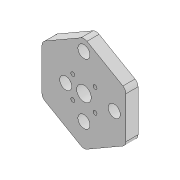
# Autodesk Inventor part: Flange
Saved by Autodesk Inventor 2020 (Build 240168000, 168)
## iProperties
Created: 2021-08-17
Part Number: Flange
Material: 一般
Document SubType Name: Modeling
Designer: ken113
Density: 1 g/cm^3
Appearance: 既定
Author: ken113
Autodesk Inventor part; units mm, degrees
ref_plane "YZ Plane" through (0, 0, 0) normal (1, 0, 0) x (0, 1, 0)
ref_plane "XZ Plane" through (0, 0, 0) normal (0, 1, 0) x (-1, 0, 0)
ref_plane "XY Plane" through (0, 0, 0) normal (0, 0, 1) x (1, 0, 0)
sketch "スケッチ1" plane through (0, 0, 0) normal (0, 0, 1) x (1, 0, 0)
  line L0 (0, 40) -> (34.641, 20)
  line L1 (34.641, 20) -> (34.641, -20)
  line L2 (34.641, -20) -> (0, -40)
  line L3 (0, -40) -> (-34.641, -20)
  line L4 (-34.641, -20) -> (-34.641, 20)
  line L5 (-34.641, 20) -> (0, 40)
  point P0 (0, 0)
  point P1 (0, 0)
  dimension "d0" = 40
  constraints: 12 end point, 1 coincident, 1 vertical alignment, 13 other
  measures "d0" distance of point (0, 0) L0.start
extrude "押し出し1" add sketch "スケッチ1" along normal blind 10
sketch "スケッチ2" plane through (0, 0, 10) normal (0, 0, 1) x (1, 0, 0)
  line L0 (0, -40) -> (34.641, -20) projected
  line L1 (34.641, -20) -> (34.641, 20) projected
  line L2 (34.641, 20) -> (0, 40) projected
  line L3 (0, 40) -> (-34.641, 20) projected
  line L4 (-34.641, 20) -> (-34.641, -20) projected
  line L5 (-34.641, -20) -> (0, -40) projected
  point P0 (0, 0)
  point P1 (0, 30)
  point P2 (25, 0)
  point P3 (0, -20)
  point P4 (-15, 0)
  dimension "d3" = 30
  dimension "d4" = 25
  dimension "d5" = 20
  dimension "d6" = 15
  measures "d3" distance of point (0, 30) point (0, 0)
  measures "d4" distance of point (25, 0) point (0, 0)
  measures "d5" distance of point (0, -20) point (0, 0)
  measures "d6" distance of point (0, 0) point (-15, 0)
hole "穴1" at (0, 30, 10) at (25, 0, 10) at (0, -20, 10) at (-15, 0, 10) direction (0, 0, -1) diameter 4.2 depth 10 counterbore diameter 10 counterbore depth 7
sketch "スケッチ3" plane through (0, 0, 0) normal (0, 0, -1) x (-1, 0, 0)
  circle A0 centre (0, -20) radius 2.1 projected
  circle A1 centre (0, 30) radius 2.1 projected
  circle A2 centre (-25, 0) radius 2.1 projected
  circle A3 centre (15, 0) radius 2.1 projected
  line L0 (0, -40) -> (-34.641, -20) projected
  line L1 (34.641, -20) -> (0, -40) projected
  line L2 (34.641, 20) -> (34.641, -20) projected
  line L3 (0, 40) -> (34.641, 20) projected
  line L4 (-34.641, 20) -> (0, 40) projected
  line L5 (-34.641, -20) -> (-34.641, 20) projected
  circle A4 centre (0, 0) radius 13
  point P0 (9.1924, -9.1924)
  point P1 (9.1924, 9.1924)
  point P2 (-9.1924, 9.1924)
  point P3 (-9.1924, -9.1924)
  dimension "d14" = 26
  dimension "d17" = 360
  constraints: 1 coincident, 1 horizontal alignment, 8 other
hole "穴2" at (-9.1924, -9.1924, 0) at (-9.1924, 9.1924, 0) at (9.1924, 9.1924, 0) at (9.1924, -9.1924, 0) direction (0, 0, 1) diameter 3.242 depth 12 thread size "M4x0.7" class "6H" standard "ISO Metric profile"
sketch "スケッチ4" plane through (0, 0, 0) normal (0, 0, -1) x (-1, 0, 0)
  circle A0 centre (-9.1924, 9.1924) radius 1.621 projected
  circle A1 centre (9.1924, -9.1924) radius 1.621 projected
  circle A2 centre (9.1924, 9.1924) radius 1.621 projected
  circle A3 centre (-9.1924, -9.1924) radius 1.621 projected
  circle A4 centre (0, -20) radius 2.1 projected
  circle A5 centre (0, 30) radius 2.1 projected
  circle A6 centre (-25, 0) radius 2.1 projected
  circle A7 centre (15, 0) radius 2.1 projected
  line L0 (0, -40) -> (-34.641, -20) projected
  line L1 (34.641, -20) -> (0, -40) projected
  line L2 (34.641, 20) -> (34.641, -20) projected
  line L3 (0, 40) -> (34.641, 20) projected
  line L4 (-34.641, 20) -> (0, 40) projected
  line L5 (-34.641, -20) -> (-34.641, 20) projected
  point P0 (0, 0)
hole "穴3" at (0, 30, 0) at (-15, 0, 0) at (0, -20, 0) at (25, 0, 0) direction (0, 0, 1) diameter 5.5 depth 12 countersink diameter 10.6 countersink angle 90
sketch "スケッチ5" plane through (0, 0, 0) normal (0, 0, -1) x (-1, 0, 0)
  circle A0 centre (0, 0) radius 6
  dimension "d33" = 12
  constraints: 1 centre point, 1 coincident
  measures "d33" diameter of A0
extrude "押し出し2" cut sketch "スケッチ5" against normal blind 10
fillet "フィレット1" radius 5 6 edges at (0, 40, 5) (-34.641, 20, 5) (-34.641, -20, 5) (0, -40, 5) (34.641, -20, 5) (34.641, 20, 5)
